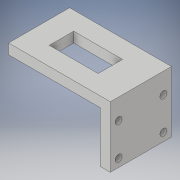
# Autodesk Inventor part: L-Halterung Servo
Saved by Autodesk Inventor 2018 (Build 220112000, 112)
## iProperties
Created: 2018-01-26
Part Number: L-Halterung Servo
Material: Generisch
Document SubType Name: Modeling
Designer: fhinstall
Density: 1 g/cm^3
Appearance: Vorgabe
Author: fhinstall
Autodesk Inventor part; units mm, degrees
ref_plane "YZ Plane" through (0, 0, 0) normal (1, 0, 0) x (0, 1, 0)
ref_plane "XZ Plane" through (0, 0, 0) normal (0, 1, 0) x (-1, 0, 0)
ref_plane "XY Plane" through (0, 0, 0) normal (0, 0, 1) x (1, 0, 0)
sketch "Skizze1" plane through (0, 0, 0) normal (0, 1, 0) x (-1, 0, 0)
  line L0 (50, 5.2632) -> (0, 5.2632)
  line L1 (0, 5.2632) -> (0, -24.7368)
  line L2 (0, -24.7368) -> (5, -24.7368)
  line L3 (5, -24.7368) -> (5, 0.2632)
  line L4 (5, 0.2632) -> (50, 0.2632)
  line L5 (50, 0.2632) -> (50, 5.2632)
  point P0 (0, 0)
  dimension "d0" = 5
  dimension "d1" = 5
  dimension "d2" = 30
  dimension "d5" = 50
  constraints: 12 end point, 4 perpendicular, 2 horizontal
  measures "d0" distance of L4.end L0.start
  measures "d1" distance of L1.end L2.end
  measures "d2" distance of L0.end L1.end
  measures "d5" distance of L0.start L0.end
extrude "Extrusion1" add sketch "Skizze1" along normal blind 30
sketch "Skizze2" plane through (-50, 0, 5.2632) normal (0, 0, 1) x (1, 0, 0)
  line L0 (11, 9) -> (35, 9)
  line L1 (35, 9) -> (35, 21)
  line L2 (35, 21) -> (11, 21)
  line L3 (11, 21) -> (11, 9)
  line L4 (50, 0) -> (50, 30) projected
  line L5 (0, 30) -> (50, 30) projected
  dimension "d6" = 15
  dimension "d7" = 24
  dimension "d8" = 12
  dimension "d9" = 9
  constraints: 8 end point, 2 parallel, 1 horizontal, 1 perpendicular
  measures "d6" distance between parallel lines of L1 L4
  measures "d7" distance of L1.end L2.end
  measures "d8" distance of L2.end L0.start
  measures "d9" distance between parallel lines of L5 L2
extrude "Extrusion2" cut sketch "Skizze2" against normal blind 5
sketch "Skizze3" plane through (0, 0, 5.2632) normal (1, 0, 0) x (0, 0, -1)
  circle A0 centre (10, 4) radius 1.7
  circle A1 centre (26, 4) radius 1.7
  circle A2 centre (10, 26) radius 1.7
  circle A3 centre (26, 26) radius 1.7
  line L0 (0, 0) -> (0, 30) projected
  line L1 (0, 30) -> (30, 30) projected
  line L2 (30, 0) -> (30, 30) projected
  point P0 (5.2632, 0)
  dimension "d12" = 3.4
  dimension "d13" = 3.4
  dimension "d14" = 3.4
  dimension "d15" = 3.4
  dimension "d16" = 10
  dimension "d17" = 22
  dimension "d18" = 4
  dimension "d19" = 10
  dimension "d20" = 4
  dimension "d21" = 22
  dimension "d22" = 4
  dimension "d23" = 4
  constraints: 4 centre point
  measures "d12" diameter of A0
  measures "d13" diameter of A2
  measures "d14" diameter of A3
  measures "d15" diameter of A1
  measures "d16" distance from line of L0 A0.centre
  measures "d17" distance of A2.centre A0.centre
  measures "d18" distance from line of L1 A2.centre
  measures "d19" distance from line of L0 A2.centre
  measures "d20" distance from line of L2 A1.centre
  measures "d21" distance of A3.centre A1.centre
  measures "d22" distance from line of L2 A3.centre
  measures "d23" distance from line of L1 A3.centre
extrude "Extrusion3" cut sketch "Skizze3" against normal blind 5
sketch "Skizze4" plane through (0, 0, 5.2632) normal (1, 0, 0) x (0, 0, -1)
  point P0 (5.2632, 0)
